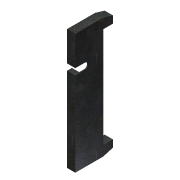
# Autodesk Inventor part: Right Side
Saved by Autodesk Inventor 2016 (Build 200138000, 138)
## iProperties
Created: 2015-05-19
Part Number: Right Side
Material: Steel
Document SubType Name: Modeling
Designer: Andy
Density: 7.85 g/cm^3
Appearance: Plate
Mass: 981.072 g
Surface Area: 496.1 cm^2
Volume: 124.977 cm^3
Author: Andy
Autodesk Inventor part; units mm, degrees
ref_plane "YZ Plane" through (0, 0, 0) normal (1, 0, 0) x (0, 1, 0)
ref_plane "XZ Plane" through (0, 0, 0) normal (0, 1, 0) x (-1, 0, 0)
ref_plane "XY Plane" through (0, 0, 0) normal (0, 0, 1) x (1, 0, 0)
sketch "Sketch1" plane through (0, 0, 0) normal (1, 0, 0) x (0, 1, 0)
  line L0 (0, 0) -> (58, 0)
  line L1 (58, -250) -> (0, -250)
  line L2 (78, -6) -> (78, -21)
  line L3 (78, -21) -> (58, -21)
  line L4 (58, -21) -> (58, -125)
  line L5 (78, -21) -> (78, -6)
  line L6 (78, -21) -> (78, -6)
  line L7 (78, -229) -> (58, -229)
  line L8 (58, -229) -> (58, -125)
  line L9 (78, -244) -> (58, -250)
  line L10 (78, -244) -> (78, -229)
  line L11 (0, 0) -> (0, -62)
  line L12 (0, -62) -> (20, -62)
  line L13 (20, -75) -> (0, -75)
  arc A0 (20, -75) -> (20, -62) centre (20, -68.5) ccw
  line L14 (78, -6) -> (78, -21)
  line L15 (78, -229) -> (78, -244)
  line L16 (0, -250) -> (0, -75)
  line L17 (0, -62) -> (0, 0)
  line L18 (58, 0) -> (0, 0)
  line L19 (0, 0) -> (0, -62)
  line L20 (0, -62) -> (20, -62)
  arc A1 (20, -75) -> (20, -62) centre (20, -68.5) ccw
  line L21 (20, -75) -> (0, -75)
  line L22 (0, -75) -> (0, -250)
  line L23 (0, -250) -> (58, -250)
  line L24 (58, 0) -> (0, 0)
  line L25 (78, -6) -> (58, 0)
  dimension "d8" = 62
  dimension "d10" = 13
  dimension "d21" = 15
  dimension "d22" = 15
  constraints: 52 end point, 7 collinear, 6 perpendicular, 5 parallel, 4 point on circle, 2 centre point, 2 horizontal, 1 coincident, 1 tangent
  measures "d8" distance of L0.start L11.end
  measures "d10" distance of L12.end L13.start
  measures "d21" distance of L9.start L7.start
  measures "d22" distance of L2.start L2.end
extrude "Extrusion2" add sketch "Sketch1" along normal blind 17
sketch "Sketch2" plane through (0, 0, 0) normal (-1, 0, 0) x (0, 0, 1)
  line L0 (-75, 0) -> (-250, 0) projected
  line L1 (-229, 42) -> (-238, 42)
  line L2 (-238, 42) -> (-238, 10)
  line L3 (-75, 0) -> (-250, 0) projected
  line L4 (-229, 42) -> (-179, 42)
  line L5 (-179, 42) -> (-179, 56)
  line L6 (-238, 10) -> (-125, 10)
  line L7 (-21, 42) -> (-12, 42)
  line L8 (-12, 42) -> (-12, 10)
  line L9 (-21, 42) -> (-71, 42)
  line L10 (-71, 42) -> (-71, 56)
  line L11 (-12, 10) -> (-125, 10)
  line L12 (-179, 56) -> (-71, 56)
  point P0 (-229, 58)
  dimension "d14" = 16
  dimension "d15" = 9
  dimension "d23" = 32
  constraints: 22 end point, 2 perpendicular, 1 horizontal
  measures "d14" distance of point (-229, 58) L1.start
  measures "d15" distance of L1.start L1.end
  measures "d23" distance between parallel lines of L6 L4
extrude "Extrusion3" cut sketch "Sketch2" against normal blind 15
body "Solid2"
